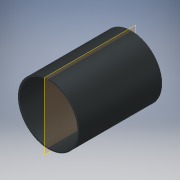
# Autodesk Inventor part: Moteur electrique
Saved by Autodesk Inventor 2018 (Build 220112000, 112)
## iProperties
Created: 2017-10-08
Part Number: Moteur electrique
Material: Iron, Cast
Document SubType Name: Modeling
Designer: liamg
Density: 7.15 g/cm^3
Appearance: Iron Gray
Author: liamg
Autodesk Inventor part; units mm, degrees
ref_plane "XZ Plane" through (0, 0, 0) normal (0, 1, 0) x (-1, 0, 0)
ref_plane "XY Plane" through (0, 0, 0) normal (0, 0, 1) x (1, 0, 0)
sketch "Sketch3" plane through (0, 0, 0) normal (0, 0, 1) x (1, 0, 0)
  circle A0 centre (0, 0) radius 17.93
  circle A1 centre (0, 0) radius 17.13
  dimension "d6" = 35.86
  dimension "d7" = 0.8
  constraints: 2 centre point, 2 coincident
  measures "d6" diameter of A0
  measures "d7" radial gap between concentric circles of A1 A0
extrude "Extrusion3" add sketch "Sketch3" along normal blind 48.94
body "Solid2"
